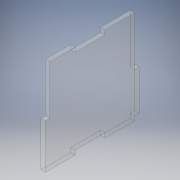
# Autodesk Inventor part: cham_side
Saved by Autodesk Inventor 2017.2 (Build 212233000, 233)
## iProperties
Created: 2017-06-02
Part Number: cham_side
Material: Generic
Document SubType Name: Modeling
Designer: SandeepSH
Density: 1 g/cm^3
Appearance: Polycarbonate - Clear
Author: SandeepSH
Autodesk Inventor part; units mm, degrees
ref_plane "YZ Plane" through (0, 0, 0) normal (1, 0, 0) x (0, 1, 0)
ref_plane "XZ Plane" through (0, 0, 0) normal (0, 1, 0) x (-1, 0, 0)
ref_plane "XY Plane" through (0, 0, 0) normal (0, 0, 1) x (1, 0, 0)
sketch "Sketch1" plane through (0, 0, 0) normal (1, 0, 0) x (0, 1, 0)
  line L0 (-31.5, 31.5) -> (31.5, 31.5)
  line L1 (31.5, 31.5) -> (31.5, -31.5)
  line L2 (31.5, -31.5) -> (-31.5, -31.5)
  line L3 (-31.5, -31.5) -> (-31.5, 31.5)
  line L4 (-31.5, 31.5) -> (31.5, -31.5) construction
  line L5 (31.5, 31.5) -> (-31.5, -31.5) construction
  line L6 (31.5, 31.5) -> (-1.5, 31.5)
  line L7 (-1.5, 31.5) -> (-1.5, 28.5)
  line L8 (-1.5, 28.5) -> (31.5, 28.5)
  line L9 (31.5, 28.5) -> (31.5, 31.5)
  line L10 (31.5, -31.5) -> (-1.5, -31.5)
  line L11 (-1.5, -31.5) -> (-1.5, -28.5)
  line L12 (-1.5, -28.5) -> (31.5, -28.5)
  line L13 (31.5, -28.5) -> (31.5, -31.5)
  line L14 (-31.5, 11.5) -> (-28.5, 11.5)
  line L15 (-28.5, 11.5) -> (-28.5, -8.5)
  line L16 (-28.5, -8.5) -> (-31.5, -8.5)
  line L17 (-31.5, -8.5) -> (-31.5, 11.5)
  line L18 (-31.5, -28.5) -> (-28.5, -28.5)
  line L19 (-28.5, -28.5) -> (-28.5, -31.5)
  line L20 (-28.5, -31.5) -> (-31.5, -31.5)
  line L21 (-31.5, -31.5) -> (-31.5, -28.5)
  line L22 (31.5, 11.5) -> (28.5, 11.5)
  line L23 (28.5, 11.5) -> (28.5, -8.5)
  line L24 (28.5, -8.5) -> (31.5, -8.5)
  line L25 (31.5, -8.5) -> (31.5, 11.5)
  point P0 (0, 0)
  dimension "d0" = 63
  dimension "d1" = 63
  dimension "d2" = 33
  dimension "d3" = 3
  dimension "d4" = 3
  dimension "d5" = 3
  dimension "d6" = 20
  dimension "d7" = 20
  dimension "d8" = 3
  constraints: 52 end point, 12 parallel, 6 horizontal, 6 perpendicular, 4 point on line, 2 midpoint, 1 collinear
  measures "d0" distance of L1.end L2.end
  measures "d1" distance of L0.end L1.end
  measures "d2" distance of L8.end L7.end
  measures "d3" distance of L7.end L6.end
  measures "d4" distance between parallel lines of L2 L12
  measures "d5" distance of L15.end L16.end
  measures "d6" distance of L14.end L15.end
  measures "d7" distance between parallel lines of L14 L0
  measures "d8" distance of L24.end L23.end
extrude "Extrusion1" add sketch "Sketch1" along normal blind 3 contours L0 L7 L8 L1 L22 L23 L24 L12 L11 L2 L19 L18 L3 L16 L15 L14
equation "\"d4\" = d3"
body "Solid1"
